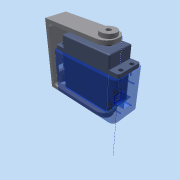
# Autodesk Inventor part: servo-mount-skull
Saved by Autodesk Inventor 2015 SP1 (Build 190203100, 203)
## iProperties
Created: 2023-12-10
Part Number: servo-mount-skull
Material: Типовые
Document SubType Name: Modeling
Designer: boss
Density: 1 g/cm^3
Appearance: По умолчанию
Author: boss
Autodesk Inventor part; units mm, degrees
ref_plane "XZ Plane" through (0, 0, 0) normal (0, 1, 0) x (-1, 0, 0)
ref_plane "XY Plane" through (0, 0, 0) normal (0, 0, 1) x (1, 0, 0)
sketch "sc-servo" plane through (0, 0, 0) normal (0, 0, 1) x (1, 0, 0)
  line L0 (-25.75, 10) -> (25.75, 10)
  line L1 (27.25, 8.5) -> (27.25, -8.5)
  line L2 (25.75, -10) -> (-25.75, -10)
  line L3 (-27.25, -8.5) -> (-27.25, 8.5)
  line L4 (-27.25, 10) -> (27.25, -10) construction
  line L5 (27.25, 10) -> (-27.25, -10) construction
  line L6 (-20, 10) -> (20, 10)
  line L7 (20, 10) -> (20, -10)
  line L8 (20, -10) -> (-20, -10)
  line L9 (-20, -10) -> (-20, 10)
  line L10 (-20, 10) -> (20, -10) construction
  line L11 (20, 10) -> (-20, -10) construction
  arc A0 (27.25, 8.5) -> (25.75, 10) centre (25.75, 8.5) ccw
  arc A1 (25.75, -10) -> (27.25, -8.5) centre (25.75, -8.5) ccw
  arc A2 (-27.25, -8.5) -> (-25.75, -10) centre (-25.75, -8.5) ccw
  arc A3 (-25.75, 10) -> (-27.25, 8.5) centre (-25.75, 8.5) ccw
  line L12 (-34.7079, 0) -> (34.7079, 0) construction
  circle A4 centre (10, 0) radius 2.95
  line L13 (24.75, -5) -> (-24.75, -5) construction
  line L14 (-24.75, -5) -> (-24.75, 5) construction
  line L15 (-24.75, 5) -> (24.75, 5) construction
  line L16 (24.75, 5) -> (24.75, -5) construction
  line L17 (24.75, -5) -> (-24.75, 5) construction
  line L18 (-24.75, -5) -> (24.75, 5) construction
  circle A5 centre (-24.75, 5) radius 1.6
  circle A6 centre (-24.75, -5) radius 1.6
  circle A7 centre (24.75, 5) radius 1.6
  circle A8 centre (24.75, -5) radius 1.6
  point P0 (0, 0)
  point P1 (0, 0)
  dimension "d0" = 54.5
  dimension "d1" = 20
  dimension "d2" = 40
  dimension "d3" = 20
  dimension "d4" = 1.5
  dimension "d5" = 5.9
  dimension "d6" = 10
  dimension "d7" = 49.5
  dimension "d8" = 10
  dimension "d9" = 3.2
  dimension "d10" = 3.2
  dimension "d11" = 3.2
  dimension "d12" = 3.2
  dimension "d22" = 17.25
  constraints: 38 end point, 9 centre point, 9 point on line, 8 midpoint, 8 point on circle, 8 tangent, 6 parallel, 4 coincident, 4 horizontal, 3 equal radius, 3 perpendicular
  measures "d0" distance of L4.end L5.end
  measures "d1" distance of L5.start L4.end
  measures "d2" distance of L7.end L8.end
  measures "d3" distance of L6.end L7.end
  measures "d4" radius of A0
  measures "d5" diameter of A4
  measures "d6" distance from line of L7 A4.centre
  measures "d7" distance of L14.end L15.end
  measures "d8" distance of L13.end L14.end
  measures "d9" diameter of A5
  measures "d10" diameter of A6
  measures "d11" diameter of A7
  measures "d12" diameter of A8
  measures "d22" horizontal distance of L1.start A4.centre
sketch "sc-servo-harness" plane through (0, 0, 0) normal (0, 0, 1) x (1, 0, 0)
  line L0 (-28, -12.75) -> (28, -12.75)
  line L1 (28, -12.75) -> (28, 12.75)
  line L2 (28, 12.75) -> (-28, 12.75)
  line L3 (-28, 12.75) -> (-28, -12.75)
  line L4 (-28, -12.75) -> (28, 12.75) construction
  line L5 (28, -12.75) -> (-28, 12.75) construction
  circle A0 centre (10, 0) radius 3
  point P0 (0, 0)
  dimension "d23" = 56
  dimension "d24" = 25.5
  dimension "d29" = 6
  constraints: 12 end point, 2 midpoint, 2 parallel, 1 centre point, 1 coincident, 1 horizontal, 1 perpendicular
  measures "d23" distance of L2.end L1.end
  measures "d24" distance of L1.end L0.end
  measures "d29" diameter of A0
extrude "Выдавливание1" add sketch "sc-servo" along normal blind 12.7 and the other way blind 27.8 contours L0 L7 L2 L9 | A4
extrude "Выдавливание2" add sketch "sc-servo" along normal blind 18.9 separate body contours A4
extrude "Выдавливание3" add sketch "sc-servo" along normal blind 3.1 contours L0 L9 L2 A2 L3 A3 | L0 A0 L1 A1 L2 L7 bodies 1
fillet "Сопряжение1" radius 1 16 edges at (20, 10, -13.9) (0, 10, -27.8) (20, 0, -27.8) (20, -10, -13.9) (20, 0, 12.7) (20, 10, 7.9) (0, -10, -27.8) (-20, 10, -13.9) (-20, 0, -27.8) (-20, 10, 7.9) (-20, 0, 12.7) (-20, -10, 7.9) (0, -10, 12.7) (0, 10, 12.7) (20, -10, 7.9) (-20, -10, -13.9)
extrude "Выдавливание4" add sketch "sc-servo-harness" against normal blind 32 separate body contours L3 L2 L1 L0 | A0
extrude "Выдавливание6" add sketch "sc-servo-harness" against normal blind 36 contours A0 bodies 3
extrude "Выдавливание5" cut sketch "sc-servo" against normal blind 28.5 contours L0 L7 L2 L9 | A4 bodies 3
hole "Отверстие1" at (-24.75, 5, 0) at (-24.75, -5, 0) at (24.75, -5, 0) at (24.75, 5, 0) direction (0, 0, -1) diameter 1 depth 5 bodies 3
sketch "Эскиз3" plane through (0, 0, 0) normal (0, 1, 0) x (-1, 0, 0)
  line L0 (-7.05, 18.9) -> (-12.95, 18.9) projected
  line L1 (-12.95, 0) -> (-7.05, 0) projected
  line L2 (-13, -36) -> (-7, -36) projected
  line L3 (-7, -32) -> (-13, -32) projected
  line L4 (-28, 0) -> (28, 0) projected
  line L5 (-17, 18.4) -> (38, 18.4)
  line L6 (38, 18.4) -> (38, 15.4)
  line L7 (38, 15.4) -> (-17, 15.4)
  line L8 (-17, 15.4) -> (-17, 18.4)
  line L9 (38, 18.4) -> (35, 18.4)
  line L10 (35, 18.4) -> (35, -36.5)
  line L11 (35, -36.5) -> (38, -36.5)
  line L12 (38, -36.5) -> (38, 18.4)
  line L13 (-17, -33.5) -> (38, -33.5)
  line L14 (38, -33.5) -> (38, -36.5)
  line L15 (38, -36.5) -> (-17, -36.5)
  line L16 (-17, -36.5) -> (-17, -33.5)
  line L17 (-28, 0) -> (28, 0) construction
  line L18 (-28, 0) -> (-28, -32) construction
  line L19 (28, -32) -> (-28, -32) construction
  line L20 (28, 0) -> (28, -32) construction
  line L21 (20, 3.1) -> (20, 11.7) construction
  line L22 (19, 12.7) -> (-19, 12.7) construction
  point P0 (0, 0)
  point P1 (0, 0)
  dimension "d40" = 2.7
  dimension "d41" = 3
  dimension "d42" = 55
  dimension "d43" = 18
  dimension "d44" = 3
  dimension "d45" = 3
  dimension "d46" = 1.5
  constraints: 24 end point, 6 parallel, 3 horizontal, 3 perpendicular, 1 midpoint, 1 point on line
  measures "d40" distance between parallel lines of L22 L7
  measures "d41" distance between parallel lines of L5 L7
  measures "d42" distance of L5.start L5.end
  measures "d43" distance between parallel lines of L12 L21
  measures "d44" distance between parallel lines of L12 L10
  measures "d45" distance between parallel lines of L15 L13
  measures "d46" distance between parallel lines of L19 L13
extrude "Выдавливание7" add sketch "Эскиз3" along normal mid plane 18 separate body
sketch "Эскиз4" plane through (-38, -9, 18.4) normal (0, 0, 1) x (1, 0, 0)
  circle A0 centre (48, 9) radius 2.95 projected
  circle A1 centre (48, 9) radius 1.95
  circle A2 centre (48, 9) radius 5.95
  point P0 (38, 9)
  dimension "d49" = 1
  dimension "d50" = 3
  constraints: 2 centre point
  measures "d49" radial gap between concentric circles of A0 A1
  measures "d50" radial gap between concentric circles of A0 A2
extrude "Выдавливание8" add sketch "Эскиз4" along normal blind 3 contours A0 | A2 bodies 4
extrude "Выдавливание9" cut sketch "Эскиз4" against normal through all contours A0 | A1 bodies 4
sketch "Эскиз5" plane through (17, 9, -36.5) normal (0, 0, -1) x (-1, 0, 0)
  circle A0 centre (7, -9) radius 3 projected
  circle A1 centre (7, -9) radius 4
  circle A2 centre (7, -9) radius 6
  point P0 (17, -9)
  dimension "d55" = 1
  dimension "d56" = 2
  constraints: 2 centre point
  measures "d55" radial gap between concentric circles of A0 A1
  measures "d56" radial gap between concentric circles of A1 A2
extrude "Выдавливание10" add sketch "Эскиз5" along normal blind 3 contours A0 | A1 | A2 bodies 4
sketch "Эскиз6" plane through (20, -10, 0) normal (-1, 0, 0) x (0, 0, 1)
  line L0 (0, 20) -> (0, 0) construction
  line L1 (0, 20) -> (-28.5, 20) construction
  line L2 (-28.5, 20) -> (-28.5, 0) construction
  line L3 (0, 0) -> (-28.5, 0) construction
  line L4 (-77.4346, 10) -> (20.4346, 10) construction
  line L5 (-28.5, 20) -> (-28.5, 0) projected
  line L6 (-24.5, 13.3) -> (-18.5, 13.3)
  line L7 (-18.5, 13.3) -> (-18.5, 6.7)
  line L8 (-18.5, 6.7) -> (-24.5, 6.7)
  line L9 (-24.5, 6.7) -> (-24.5, 13.3)
  line L10 (-24.5, 13.3) -> (-18.5, 6.7) construction
  line L11 (-18.5, 13.3) -> (-24.5, 6.7) construction
  point P0 (0, 10)
  point P1 (-28.5, 10)
  point P2 (-21.5, 10)
  dimension "d59" = 4
  dimension "d60" = 10
  dimension "d61" = 6.6
  constraints: 14 end point, 4 midpoint, 2 horizontal, 2 parallel, 1 perpendicular, 1 point on line
  measures "d59" distance between parallel lines of L2 L9
  measures "d60" distance between parallel lines of L2 L7
  measures "d61" distance between parallel lines of L8 L6
extrude "Выдавливание11" cut sketch "Эскиз6" against normal through all bodies 3
fillet "Сопряжение2" radius 4 4 edges at (28, 12.75, -16) (-28, 12.75, -16) (-28, -12.75, -16) (28, -12.75, -16)
ref_plane "РабПлоскость1" through (-38, 0, 0) normal (1, 0, 0) x (0, 1, 0)
sketch "Эскиз8" plane through (-38, 0, 0) normal (1, 0, 0) x (0, 1, 0)
  line L0 (0, 38.2561) -> (0, -38.2561) construction
  line L1 (5.5, -27) -> (-5.5, -27) construction
  line L2 (-5.5, -27) -> (-5.5, -10) construction
  line L3 (-5.5, -10) -> (5.5, -10) construction
  line L4 (5.5, -10) -> (5.5, -27) construction
  line L5 (5.5, -27) -> (-5.5, -10) construction
  line L6 (-5.5, -27) -> (5.5, -10) construction
  point P0 (0, 0)
  point P1 (0, 0)
  point P2 (0, -18.5)
  dimension "d66" = 17
  dimension "d67" = 10
  dimension "d68" = 11
  constraints: 14 end point, 5 coincident, 3 midpoint, 2 parallel, 1 horizontal, 1 perpendicular, 1 point on line, 1 vertical
  measures "d66" distance of L1.end L2.end
  measures "d67" distance from line of point (0, 0) L3
  measures "d68" distance of L2.end L3.end
hole "Отверстие2" at (-38, 5.5, -10) at (-38, -5.5, -10) at (-38, -5.5, -27) at (-38, 5.5, -27) direction (1, 0, 0) diameter 1 depth 80 countersink diameter 1.5 countersink angle 90 bodies 4 3
extrude "Выдавливание12" cut sketch "Эскиз6" along normal through all bodies 4
hole "Отверстие3" at (-33, 0, -36.5) direction (0, 0, 1) diameter 8.5 depth 8 bodies 4
fillet "Сопряжение3" radius 3 2 edges at (-35, 6.375, -33.5) (-35, -6.375, -33.5)
fillet "Сопряжение4" radius 8 4 edges at (17, 9, 16.9) (17, -9, 16.9) (17, 9, -35) (17, -9, -35)
fillet "Сопряжение5" radius 3 1 edges at (-35, 0, 15.4)
equation "\"servaBodyHeght\" = 40.5"
